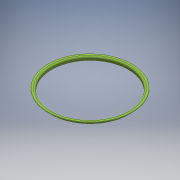
# Autodesk Inventor part: кол_062
Saved by Autodesk Inventor 2016 (Build 200138000, 138)
## iProperties
Created: 2021-05-03
Part Number: кол_062
Material: Типовые
Document SubType Name: Modeling
Designer: Лол
Density: 1 g/cm^3
Appearance: Оливково-зеленый
Author: Лол
Autodesk Inventor part; units mm, degrees
ref_plane "YZ Plane" through (0, 0, 0) normal (1, 0, 0) x (0, 1, 0)
ref_plane "XZ Plane" through (0, 0, 0) normal (0, 1, 0) x (-1, 0, 0)
ref_plane "XY Plane" through (0, 0, 0) normal (0, 0, 1) x (1, 0, 0)
sketch "Эскиз1" plane through (0, 0, 0) normal (1, 0, 0) x (0, 1, 0)
  line L0 (-6.86, 0) -> (41.16, 0) construction
  line L1 (0, 0.66) -> (0, -3.96) construction
  line L2 (34.3, 0) -> (31, 0)
  line L3 (31, -3.3) -> (34.3, 0)
  line L4 (31, -3.3) -> (31, 0)
  point P0 (0, 0)
  dimension "d0" = 31
  dimension "d1" = 3.3
  dimension "d2" = 45
  constraints: 6 end point, 2 point on line, 1 perpendicular
  measures "d0" distance between parallel lines of L1 L4
  measures "d1" distance of L2.end L3.start
  measures "d2" angle of L3 L4
revolve "Вращение1" add sketch "Эскиз1" angle 360 about axis through (0, 0, 0) along (0, 0, -1)
fillet "Сопряжение1" radius 1.3 1 edges at (0, -31, 0)
fillet "Сопряжение2" radius 0.25 1 edges at (0, -34.3, 0)
fillet "Сопряжение3" radius 0.25 1 edges at (0, -31, -3.3)
